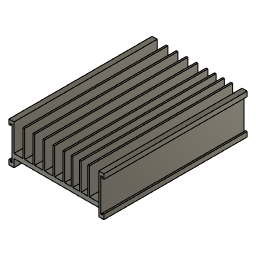
heatsink v3 (Autodesk Fusion 360 design; units mm, degrees)
Autodesk Fusion 360 part; units mm, degrees
sketch "Sketch1" plane through (0, 0, 0) normal (0, 1, 0) x (1, 0, 0)
  line L0 (-26.4331, -0.9293) -> (27.0669, -0.9293)
  line L1 (27.0669, -0.9293) -> (27.0669, 1.8707)
  line L2 (27.0669, 1.8707) -> (-26.4331, 1.8707)
  line L3 (-26.4331, 1.8707) -> (-26.4331, -0.9293)
  point P0 (-26.4331, -0.9293)
  dimension "d1" = 53.5
  dimension "d2" = 2.8
  constraint horizontal L0
  constraint vertical L1
  constraint horizontal L2
  constraint vertical L3
  constraint coincident P0 L0.start
  measures "d1" distance of P0 L0.end
  measures "d2" distance of P0 L2.end
sketch "Sketch2" plane through (0.0669, 0, -0.4707) normal (0, 1, 0) x (1, 0, 0)
sketch "Sketch3" plane through (0, 0, 0) normal (0, 1, 0) x (1, 0, 0)
  line L0 (-20.7, -0.9) -> (-19.7, -0.9)
  line L1 (-19.7, -0.9) -> (-19.7, -17.9)
  line L2 (-19.7, -17.9) -> (-20.7, -17.9)
  line L3 (-20.7, -17.9) -> (-20.7, -0.9)
  line L4 (-13.4, -17.9) -> (-14.4, -17.9)
  line L5 (-13.4, -0.9) -> (-13.4, -17.9)
  line L6 (-14.4, -17.9) -> (-14.4, -0.9)
  line L7 (-14.4, -0.9) -> (-13.4, -0.9)
  line L8 (-7.1, -17.9) -> (-8.1, -17.9)
  line L9 (-7.1, -0.9) -> (-7.1, -17.9)
  line L10 (-8.1, -17.9) -> (-8.1, -0.9)
  line L11 (-8.1, -0.9) -> (-7.1, -0.9)
  line L12 (-0.8, -17.9) -> (-1.8, -17.9)
  line L13 (-0.8, -0.9) -> (-0.8, -17.9)
  line L14 (-1.8, -17.9) -> (-1.8, -0.9)
  line L15 (-1.8, -0.9) -> (-0.8, -0.9)
  line L16 (5.5, -17.9) -> (4.5, -17.9)
  line L17 (5.5, -0.9) -> (5.5, -17.9)
  line L18 (4.5, -17.9) -> (4.5, -0.9)
  line L19 (4.5, -0.9) -> (5.5, -0.9)
  line L20 (9.7, -17.9) -> (9.7, -0.9)
  line L21 (9.7, -0.9) -> (10.7, -0.9)
  line L22 (10.7, -0.9) -> (10.7, -17.9)
  line L23 (10.7, -17.9) -> (9.7, -17.9)
  line L24 (14.9, -17.9) -> (14.9, -0.9)
  line L25 (14.9, -0.9) -> (15.9, -0.9)
  line L26 (15.9, -0.9) -> (15.9, -17.9)
  line L27 (15.9, -17.9) -> (14.9, -17.9)
  line L28 (20.1, -17.9) -> (20.1, -0.9)
  line L29 (20.1, -0.9) -> (21.1, -0.9)
  line L30 (21.1, -0.9) -> (21.1, -17.9)
  line L31 (21.1, -17.9) -> (20.1, -17.9)
  line L32 (-26.43, 6.88) -> (-27.63, 6.88)
  line L33 (-27.63, 6.88) -> (-27.63, -18.12)
  line L34 (-27.63, -18.12) -> (-26.43, -18.12)
  line L35 (-26.43, -18.12) -> (-26.43, 6.88)
  line L36 (-27.63, 6.88) -> (-29.63, 6.88)
  line L37 (-29.63, 6.88) -> (-29.63, 4.88)
  line L38 (-29.63, 4.88) -> (-27.63, 4.88)
  line L39 (-27.63, 4.88) -> (-27.63, 6.88)
  line L40 (-29.63, 4.88) -> (-28.63, 4.88)
  line L41 (-28.63, 4.88) -> (-28.63, 3.88)
  line L42 (-28.63, 3.88) -> (-29.63, 3.88)
  line L43 (-29.63, 3.88) -> (-29.63, 4.88)
  line L44 (-27.63, -18.12) -> (-29.63, -18.12)
  line L45 (-29.63, -18.12) -> (-29.63, -16.12)
  line L46 (-29.63, -16.12) -> (-27.63, -16.12)
  line L47 (-27.63, -16.12) -> (-27.63, -18.12)
  line L48 (-29.63, -16.12) -> (-28.63, -16.12)
  line L49 (-28.63, -16.12) -> (-28.63, -15.12)
  line L50 (-28.63, -15.12) -> (-29.63, -15.12)
  line L51 (-29.63, -15.12) -> (-29.63, -16.12)
  line L52 (-27.63, 6.88) -> (-29.63, 6.88)
  line L53 (-27.63, -16.12) -> (-27.63, -18.12)
  line L54 (-29.63, -15.12) -> (-29.63, -16.12)
  line L55 (-27.63, 6.88) -> (-27.63, -18.12)
  line L56 (-29.63, -18.12) -> (-29.63, -16.12)
  line L57 (-29.63, 3.88) -> (-29.63, 4.88)
  line L58 (-27.63, -18.12) -> (-26.43, -18.12)
  line L59 (-28.63, -16.12) -> (-28.63, -15.12)
  line L60 (-29.63, -16.12) -> (-28.63, -16.12)
  line L61 (-29.63, -16.12) -> (-27.63, -16.12)
  line L62 (-26.43, -18.12) -> (-26.43, 6.88)
  line L63 (-29.63, 4.88) -> (-27.63, 4.88)
  line L64 (-26.43, 6.88) -> (-27.63, 6.88)
  line L65 (-28.63, -15.12) -> (-29.63, -15.12)
  line L66 (-28.63, 4.88) -> (-28.63, 3.88)
  line L67 (-27.63, -18.12) -> (-29.63, -18.12)
  line L68 (-29.63, 4.88) -> (-28.63, 4.88)
  line L69 (-27.63, 4.88) -> (-27.63, 6.88)
  line L70 (-29.63, 6.88) -> (-29.63, 4.88)
  line L71 (-28.63, 3.88) -> (-29.63, 3.88)
  line L72 (-27.63, 4.88) -> (-27.63, 6.88)
  line L73 (-29.63, 4.88) -> (-27.63, 4.88)
  line L74 (-27.63, 6.88) -> (-29.63, 6.88)
  line L75 (-29.63, 3.88) -> (-29.63, 4.88)
  line L76 (-29.63, 6.88) -> (-29.63, 4.88)
  line L77 (-26.43, 6.88) -> (-27.63, 6.88)
  line L78 (-29.63, 6.88) -> (-29.63, 4.88)
  line L79 (-28.63, 4.88) -> (-28.63, 3.88)
  line L80 (-27.63, 6.88) -> (-29.63, 6.88)
  line L81 (-29.63, 4.88) -> (-27.63, 4.88)
  line L82 (-28.63, 4.88) -> (-28.63, 3.88)
  line L83 (-29.63, -16.12) -> (-27.63, -16.12)
  line L84 (-29.63, 4.88) -> (-28.63, 4.88)
  line L85 (-29.63, -16.12) -> (-28.63, -16.12)
  line L86 (-27.63, 4.88) -> (-27.63, 6.88)
  line L87 (-29.63, 3.88) -> (-29.63, 4.88)
  line L88 (-29.63, -15.12) -> (-29.63, -16.12)
  line L89 (-28.63, 3.88) -> (-29.63, 3.88)
  line L90 (-29.63, -15.12) -> (-29.63, -16.12)
  line L91 (-29.63, 4.88) -> (-28.63, 4.88)
  line L92 (-26.43, 6.88) -> (-27.63, 6.88)
  line L93 (-28.63, 3.88) -> (-29.63, 3.88)
  line L94 (-29.63, -16.12) -> (-27.63, -16.12)
  line L95 (-26.43, -18.12) -> (-26.43, 6.88)
  line L96 (-28.63, -16.12) -> (-28.63, -15.12)
  line L97 (-28.63, -16.12) -> (-28.63, -15.12)
  line L98 (-27.63, -16.12) -> (-27.63, -18.12)
  line L99 (-27.63, -18.12) -> (-29.63, -18.12)
  line L100 (-27.63, 6.88) -> (-27.63, -18.12)
  line L101 (-28.63, -15.12) -> (-29.63, -15.12)
  line L102 (-28.63, -15.12) -> (-29.63, -15.12)
  line L103 (-26.43, -18.12) -> (-26.43, 6.88)
  line L104 (-29.63, -16.12) -> (-28.63, -16.12)
  line L105 (-29.63, -18.12) -> (-29.63, -16.12)
  line L106 (-27.63, -18.12) -> (-26.43, -18.12)
  line L107 (-27.63, -16.12) -> (-27.63, -18.12)
  line L108 (-27.63, -18.12) -> (-26.43, -18.12)
  line L109 (-29.63, -18.12) -> (-29.63, -16.12)
  line L110 (-27.63, -18.12) -> (-29.63, -18.12)
  line L111 (-27.63, 6.88) -> (-27.63, -18.12)
  line L112 (28.27, 6.88) -> (27.07, 6.88)
  line L113 (28.27, 6.88) -> (27.07, 6.88)
  line L114 (28.27, 6.88) -> (27.07, 6.88)
  line L115 (28.27, 6.88) -> (27.07, 6.88)
  line L116 (27.07, 4.88) -> (27.07, 6.88)
  line L117 (27.07, 4.88) -> (27.07, 6.88)
  line L118 (27.07, -18.12) -> (28.27, -18.12)
  line L119 (27.07, -16.12) -> (27.07, -18.12)
  line L120 (28.27, -18.12) -> (28.27, 6.88)
  line L121 (28.27, -18.12) -> (28.27, 6.88)
  line L122 (27.07, -16.12) -> (27.07, -18.12)
  line L123 (28.27, -18.12) -> (28.27, 6.88)
  line L124 (27.07, 6.88) -> (27.07, -18.12)
  line L125 (27.07, -18.12) -> (28.27, -18.12)
  line L126 (28.27, -18.12) -> (28.27, 6.88)
  line L127 (27.07, 6.88) -> (27.07, -18.12)
  line L128 (27.07, -16.12) -> (27.07, -18.12)
  line L129 (27.07, 4.88) -> (27.07, 6.88)
  line L130 (27.07, 6.88) -> (27.07, -18.12)
  line L131 (27.07, 6.88) -> (27.07, -18.12)
  line L132 (27.07, -18.12) -> (28.27, -18.12)
  line L133 (27.07, 4.88) -> (27.07, 6.88)
  line L134 (27.07, -18.12) -> (28.27, -18.12)
  line L135 (27.07, -16.12) -> (27.07, -18.12)
  line L136 (28.27, -18.12) -> (30.27, -18.12)
  line L137 (30.27, -18.12) -> (30.27, -16.12)
  line L138 (30.27, -16.12) -> (28.27, -16.12)
  line L139 (28.27, -16.12) -> (28.27, -18.12)
  line L140 (30.27, -16.12) -> (29.27, -16.12)
  line L141 (29.27, -16.12) -> (29.27, -15.12)
  line L142 (29.27, -15.12) -> (30.27, -15.12)
  line L143 (30.27, -15.12) -> (30.27, -16.12)
  line L144 (28.27, 6.88) -> (30.27, 6.88)
  line L145 (30.27, 6.88) -> (30.27, 4.88)
  line L146 (30.27, 4.88) -> (28.27, 4.88)
  line L147 (28.27, 4.88) -> (28.27, 6.88)
  line L148 (30.27, 4.88) -> (29.27, 4.88)
  line L149 (29.27, 4.88) -> (29.27, 3.88)
  line L150 (29.27, 3.88) -> (30.27, 3.88)
  line L151 (30.27, 3.88) -> (30.27, 4.88)
  dimension "d5" = 1
  dimension "d6" = 17
  dimension "d9" = 25.2
  dimension "d10" = 0
  dimension "d13" = 15.6
  dimension "d14" = 0
  dimension "d15" = 1.2
  dimension "d16" = 25
  dimension "d17" = 2
  dimension "d18" = 2
  dimension "d19" = 1
  dimension "d20" = 1
  dimension "d21" = 2
  dimension "d22" = 2
  dimension "d23" = 1
  dimension "d24" = 1
  dimension "d25" = 1.2
  dimension "d26" = 25
  dimension "d27" = 2
  dimension "d28" = 2
  dimension "d29" = 1
  dimension "d30" = 1
  dimension "d31" = 2
  dimension "d32" = 2
  dimension "d33" = 1
  dimension "d34" = 1
  dimension "d35" = 1.2
  dimension "d36" = 25
  dimension "d37" = 2
  dimension "d38" = 2
  dimension "d39" = 1
  dimension "d40" = 1
  dimension "d41" = 2
  dimension "d42" = 2
  dimension "d43" = 1
  dimension "d44" = 1
  dimension "d45" = 1.2
  dimension "d46" = 25
  dimension "d47" = 2
  dimension "d48" = 2
  dimension "d49" = 1
  dimension "d50" = 1
  dimension "d51" = 2
  dimension "d52" = 2
  dimension "d53" = 1
  dimension "d54" = 1
  dimension "d55" = 1.2
  dimension "d56" = 25
  dimension "d58" = 2
  dimension "d62" = 2
  dimension "d65" = 1.2
  dimension "d66" = 25
  dimension "d68" = 2
  dimension "d72" = 2
  dimension "d75" = 1.2
  dimension "d76" = 25
  dimension "d78" = 2
  dimension "d82" = 2
  dimension "d85" = 1.2
  dimension "d86" = 25
  dimension "d88" = 2
  dimension "d92" = 2
  dimension "d95" = 2
  dimension "d96" = 2
  dimension "d97" = 1
  dimension "d98" = 1
  dimension "d99" = 2
  dimension "d100" = 2
  dimension "d101" = 1
  dimension "d102" = 1
  constraint horizontal L0
  constraint vertical L1
  constraint horizontal L2
  constraint vertical L3
  constraint horizontal L32
  constraint vertical L33
  constraint horizontal L34
  constraint vertical L35
  constraint horizontal L36
  constraint vertical L37
  constraint horizontal L38
  constraint vertical L39
  constraint horizontal L40
  constraint vertical L41
  constraint horizontal L42
  constraint vertical L43
  constraint horizontal L44
  constraint vertical L45
  constraint horizontal L46
  constraint vertical L47
  constraint horizontal L48
  constraint vertical L49
  constraint horizontal L50
  constraint vertical L51
  constraint horizontal L64
  constraint vertical L55
  constraint horizontal L58
  constraint vertical L62
  constraint horizontal L52
  constraint vertical L70
  constraint horizontal L63
  constraint vertical L69
  constraint horizontal L68
  constraint vertical L66
  constraint horizontal L71
  constraint vertical L57
  constraint horizontal L67
  constraint vertical L56
  constraint horizontal L61
  constraint vertical L53
  constraint horizontal L60
  constraint vertical L59
  constraint horizontal L65
  constraint vertical L54
  constraint horizontal L92
  constraint vertical L111
  constraint horizontal L108
  constraint vertical L103
  constraint horizontal L80
  constraint vertical L78
  constraint horizontal L81
  constraint vertical L72
  constraint horizontal L91
  constraint vertical L82
  constraint horizontal L93
  constraint vertical L87
  constraint horizontal L99
  constraint vertical L109
  constraint horizontal L94
  constraint vertical L98
  constraint horizontal L85
  constraint vertical L96
  constraint horizontal L102
  constraint vertical L88
  constraint horizontal L77
  constraint vertical L100
  constraint horizontal L106
  constraint vertical L95
  constraint horizontal L74
  constraint vertical L76
  constraint horizontal L73
  constraint vertical L86
  constraint horizontal L84
  constraint vertical L79
  constraint horizontal L89
  constraint vertical L75
  constraint horizontal L110
  constraint vertical L105
  constraint horizontal L83
  constraint vertical L107
  constraint horizontal L104
  constraint vertical L97
  constraint horizontal L101
  constraint vertical L90
  constraint horizontal L114
  constraint vertical L124
  constraint horizontal L132
  constraint vertical L126
  constraint vertical L133
  constraint vertical L135
  constraint horizontal L112
  constraint vertical L127
  constraint horizontal L134
  constraint vertical L123
  constraint vertical L129
  constraint vertical L128
  constraint horizontal L113
  constraint vertical L130
  constraint horizontal L125
  constraint vertical L121
  constraint vertical L117
  constraint vertical L119
  constraint horizontal L115
  constraint vertical L131
  constraint horizontal L118
  constraint vertical L120
  constraint vertical L116
  constraint vertical L122
  constraint horizontal L136
  constraint vertical L137
  constraint horizontal L138
  constraint vertical L139
  constraint horizontal L140
  constraint vertical L141
  constraint horizontal L142
  constraint vertical L143
  constraint horizontal L144
  constraint vertical L145
  constraint horizontal L146
  constraint vertical L147
  constraint horizontal L148
  constraint vertical L149
  constraint horizontal L150
  constraint vertical L151
  measures "d5" distance of L0.start L0.end
  measures "d6" distance of L0.start L2.end
  measures "d15" distance of L32.start L32.end
  measures "d16" distance of L32.start L34.end
  measures "d17" distance of L32.end L36.end
  measures "d18" distance of L32.end L38.end
  measures "d19" distance of L37.end L40.end
  measures "d20" distance of L37.end L42.end
  measures "d21" distance of L33.end L44.end
  measures "d22" distance of L33.end L46.end
  measures "d23" distance of L45.end L48.end
  measures "d24" distance of L45.end L50.end
  measures "d25" distance of L32.start L32.end
  measures "d26" distance of L32.start L34.end
  measures "d27" distance of L32.end L36.end
  measures "d28" distance of L38.end L32.end
  measures "d29" distance of L37.end L40.end
  measures "d30" distance of L37.end L42.end
  measures "d31" distance of L33.end L44.end
  measures "d32" distance of L33.end L46.end
  measures "d33" distance of L48.end L45.end
  measures "d34" distance of L45.end L50.end
  measures "d35" distance of L32.start L32.end
  measures "d36" distance of L32.start L34.end
  measures "d37" distance of L32.end L36.end
  measures "d38" distance of L38.end L32.end
  measures "d39" distance of L37.end L40.end
  measures "d40" distance of L37.end L42.end
  measures "d41" distance of L33.end L44.end
  measures "d42" distance of L33.end L46.end
  measures "d43" distance of L48.end L45.end
  measures "d44" distance of L45.end L50.end
  measures "d45" distance of L32.start L32.end
  measures "d46" distance of L32.start L34.end
  measures "d47" distance of L32.end L36.end
  measures "d48" distance of L38.end L32.end
  measures "d49" distance of L37.end L40.end
  measures "d50" distance of L37.end L42.end
  measures "d51" distance of L33.end L44.end
  measures "d52" distance of L33.end L46.end
  measures "d53" distance of L48.end L45.end
  measures "d54" distance of L50.end L45.end
  measures "d55" distance of L112.start L112.end
  measures "d56" distance of L112.start L118.end
  measures "d58" distance of L116.start L112.end
  measures "d62" distance of L118.start L119.start
  measures "d65" distance of L112.start L112.end
  measures "d66" distance of L112.start L118.end
  measures "d68" distance of L116.start L112.end
  measures "d72" distance of L118.start L119.start
  measures "d75" distance of L112.end L112.start
  measures "d76" distance of L118.end L112.start
  measures "d78" distance of L116.start L112.end
  measures "d82" distance of L118.start L119.start
  measures "d85" distance of L112.end L112.start
  measures "d86" distance of L118.end L112.start
  measures "d88" distance of L116.start L112.end
  measures "d92" distance of L118.start L119.start
  measures "d95" distance of L118.end L136.end
  measures "d96" distance of L118.end L138.end
  measures "d97" distance of L137.end L140.end
  measures "d98" distance of L137.end L142.end
  measures "d99" distance of L112.start L144.end
  measures "d100" distance of L112.start L146.end
  measures "d101" distance of L145.end L148.end
  measures "d102" distance of L145.end L150.end
extrude "Extrude1" add sketch "Sketch1" sketch "Sketch3" along normal blind 90.3 of sketch 2 makes body 1 at (27.07, 30.1, 9.7867) makes body 2 at (9.2346, 30.1, -1.8707)
move_body "Move1" bodies 1 2 to x (1, 0, 0) y (0, 1, 0) z (0, 0, 1) at (0, 20, 0)
sketch "Sketch4" plane through (0, 0, 0) normal (0, 1, 0) x (1, 0, 0)
